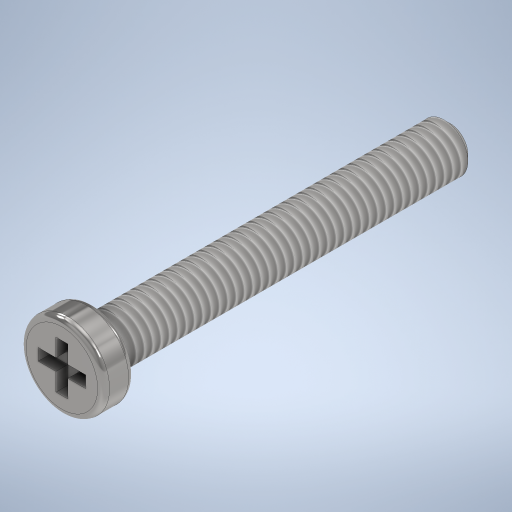
# Autodesk Inventor part: M4 16mm 십자나사
Saved by Autodesk Inventor 2023 (Build 270158000, 158)
## iProperties
Created: 2022-06-21
Part Number: M4 16mm 십자나사
Material: 일반
Document SubType Name: Modeling
Designer: user
Density: 1 g/cm^3
Appearance: 기본값
Author: user
Autodesk Inventor part; units mm, degrees
ref_plane "YZ Plane" through (0, 0, 0) normal (1, 0, 0) x (0, 1, 0)
ref_plane "XZ Plane" through (0, 0, 0) normal (0, 1, 0) x (-1, 0, 0)
ref_plane "XY Plane" through (0, 0, 0) normal (0, 0, 1) x (1, 0, 0)
sketch "스케치1" plane through (0, 0, 0) normal (0, 0, 1) x (1, 0, 0)
  circle A0 centre (0, 0) radius 3.5
  circle A1 centre (0, 0) radius 2
  dimension "d0" = 4
  dimension "d1" = 7
  constraints: 2 centre point, 2 coincident
  measures "d0" diameter of A1
  measures "d1" diameter of A0
extrude "돌출1" add sketch "스케치1" along normal blind 2.6 contours A0 | A1
extrude "돌출2" add sketch "스케치1" against normal blind 30 contours A1
fillet "모깎기1" radius 0.5 2 edges at (-3.5, 0, 0) (-3.5, 0, 2.6)
sketch "스케치2" plane through (0, 0, 2.6) normal (0, 0, 1) x (1, 0, 0)
  line L0 (-2, 0.5) -> (2, 0.5)
  line L1 (2, 0.5) -> (2, -0.5)
  line L2 (2, -0.5) -> (-2, -0.5)
  line L3 (-2, -0.5) -> (-2, 0.5)
  line L4 (-2, 0.5) -> (2, -0.5) construction
  line L5 (2, 0.5) -> (-2, -0.5) construction
  line L6 (-0.5, -2) -> (0.5, -2)
  line L7 (0.5, -2) -> (0.5, 2)
  line L8 (0.5, 2) -> (-0.5, 2)
  line L9 (-0.5, 2) -> (-0.5, -2)
  line L10 (-0.5, -2) -> (0.5, 2) construction
  line L11 (0.5, -2) -> (-0.5, 2) construction
  point P0 (0, 0)
  point P1 (-0.5, -0.5)
  point P2 (0.5, -0.5)
  point P3 (0.5, 0.5)
  point P4 (-0.5, 0.5)
  dimension "d7" = 4
  dimension "d8" = 1
  dimension "d9" = 1
  dimension "d10" = 4
  constraints: 24 end point, 4 midpoint, 4 parallel, 2 horizontal, 2 perpendicular
  measures "d7" distance of L1.end L2.end
  measures "d8" distance of L0.end L1.end
  measures "d9" distance of L8.end L7.end
  measures "d10" distance of L7.end L6.end
extrude "돌출3" cut sketch "스케치2" against normal blind 1
chamfer "모따기1" distance 0.5 angle 45 1 edges at (-2, 0, -30)
thread "스레드1" size "M4x0.7" class "6g" standard "ANSI Metric M Profile" full length
